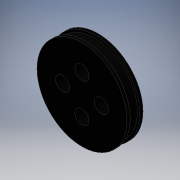
# Autodesk Inventor part: XLRotorWheel
Saved by Autodesk Inventor 2016 (Build 200138000, 138)
## iProperties
Created: 2016-03-20
Part Number: XLRotorWheel
Material: UHMW, Black
Document SubType Name: Modeling
Designer: mkepler
Density: 0.94 g/cm^3
Appearance: Smooth - Black
Mass: 2.42711 g
Surface Area: 19.4042 cm^2
Volume: 2.58204 cm^3
Author: mkepler
Autodesk Inventor part; units mm, degrees
ref_plane "YZ Plane" through (0, 0, 0) normal (1, 0, 0) x (0, 1, 0)
ref_plane "XZ Plane" through (0, 0, 0) normal (0, 1, 0) x (-1, 0, 0)
ref_plane "XY Plane" through (0, 0, 0) normal (0, 0, 1) x (1, 0, 0)
sketch "Sketch1" plane through (0, 0, 0) normal (0, 1, 0) x (-1, 0, 0)
  circle A0 centre (0, 0) radius 14
  dimension "d0" = 28
  constraints: 1 centre point, 1 coincident
  measures "d0" diameter of A0
extrude "Extrusion1" add sketch "Sketch1" along normal blind 1
sketch "Sketch2" plane through (0, 1, 0) normal (0, 1, 0) x (1, 0, 0)
  circle A0 centre (0, 0) radius 13.25
  dimension "d3" = 26.5
  constraints: 1 centre point, 1 coincident
  measures "d3" diameter of A0
extrude "Extrusion2" add sketch "Sketch2" along normal blind 3
sketch "Sketch3" plane through (0, 4, 0) normal (0, 1, 0) x (1, 0, 0)
  circle A0 centre (0, 0) radius 14
  dimension "d6" = 28
  constraints: 1 centre point, 1 coincident
  measures "d6" diameter of A0
extrude "Extrusion3" add sketch "Sketch3" along normal blind 1
sketch "Sketch4" plane through (0, 5, 0) normal (0, 1, 0) x (1, 0, 0)
  circle A0 centre (-6, 0) radius 2.2
  circle A1 centre (6, 0) radius 2.2
  circle A2 centre (0, -6) radius 2.2
  circle A3 centre (0, 6) radius 2.2
  point P0 (0, 0)
  dimension "d9" = 4.4
  dimension "d10" = 6
  dimension "d11" = 4.4
  dimension "d12" = 12
  dimension "d13" = 4.4
  dimension "d14" = 6
  dimension "d15" = 4.4
  dimension "d16" = 6
  constraints: 4 centre point
  measures "d9" diameter of A0
  measures "d10" distance of point (0, 0) A0.centre
  measures "d11" diameter of A1
  measures "d12" distance of A0.centre A1.centre
  measures "d13" diameter of A2
  measures "d14" distance of point (0, 0) A2.centre
  measures "d15" diameter of A3
  measures "d16" distance of point (0, 0) A3.centre
hole "Hole1" at (0, 5, 6) at (-6, 5, 0) at (6, 5, 0) at (0, 5, -6) direction (0, -1, 0) diameter 4.4 end through all
body "Solid1"
